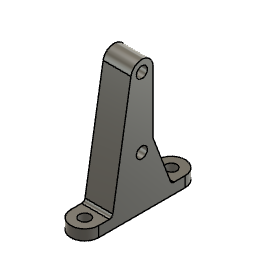
VL53L0X_Mount v9 (Autodesk Fusion 360 design; units mm, degrees)
Autodesk Fusion 360 part; units mm, degrees
sketch "Skizze1" plane through (0, 0, 0) normal (0, 1, 0) x (1, 0, 0)
  circle A0 centre (0.1472, 12.45) radius 1.6
  circle A1 centre (0.1472, -12.45) radius 1.6
  line L0 (0, 0) -> (50, 0) construction
  line L1 (4.1472, 12.45) -> (4.1472, -12.45)
  line L2 (-3.8528, 12.45) -> (-3.8528, -12.45)
  arc A2 (4.1472, 12.45) -> (-3.8528, 12.45) centre (0.1472, 12.45) ccw
  arc A3 (-3.8528, -12.45) -> (4.1472, -12.45) centre (0.1472, -12.45) ccw
  dimension "d1" = 24.9
  dimension "d2" = 3.2
  dimension "d3" = 8
  constraint coincident L0.start origin
  constraint horizontal L0
  constraint symmetric A0 A1 L0
  constraint concentric A0 A2
  constraint concentric A1 A3
  constraint symmetric L0 A2 A3
  constraint tangent L1 A3
  constraint tangent L1 A2
  constraint tangent L2 A3
  constraint vertical L2
  measures "d1" distance of A0.centre A1.centre
  measures "d2" diameter of A0
  measures "d3" diameter of A2
extrude "Extrusion1" add sketch "Skizze1" along normal blind 3
sketch "Skizze2" plane through (4.1472, 0, 0) normal (1, 0, 0) x (0, 0, -1)
  line L0 (-12.45, 0) -> (12.45, 0)
  line L1 (12.45, 0) -> (12.45, 3)
  line L2 (12.45, 3) -> (-12.45, 3)
  line L3 (-12.45, 3) -> (-12.45, 0)
  arc A0 (3.2, 35) -> (-3.1577, 35.5188) centre (0, 35) ccw
  line L4 (0, 0) -> (0, 43) construction
  circle A1 centre (0, 35) radius 1.6
  circle A2 centre (0, 15) radius 1.6
  line L5 (0, 25) -> (20, 25) construction
  line L6 (8.5, 3) -> (3.2, 17)
  line L7 (3.2, 17) -> (3.2, 35)
  line L8 (-3.1577, 35.5188) -> (-8.5, 3)
  dimension "d7" = 25
  dimension "d8" = 3.2
  dimension "d9" = 20
  dimension "d10" = 3.2
  dimension "d17" = 8.5
  dimension "d18" = 14
  dimension "d19" = 8.5
  constraint coincident L4.start origin
  constraint perpendicular L0 L4
  constraint coincident A0.centre L4
  constraint concentric A0 A1
  constraint coincident L4 A2.centre
  constraint coincident L4 L5.start
  constraint perpendicular L4 L5
  constraint symmetric A1 A2 L5
  constraint coincident L2 L6.start
  constraint tangent A0 L7
  constraint coincident L2 L8.end
  constraint tangent A0 L8
  constraint vertical L7
  measures "d7" distance of L4.start L5
  measures "d8" diameter of A1
  measures "d9" distance of A0.centre A2.centre
  measures "d10" radius of A0
  measures "d17" horizontal distance of L4.start L6.start
  measures "d18" vertical distance of L6.start L6.end
  measures "d19" horizontal distance of L4.start L8.end
extrude "Extrusion2" add sketch "Skizze2" against normal blind 8 contours L2 A0 L6 L7 L8
fillet "Abrundung3" radius 1 3 edges at (0.1472, 17, -3.2) (0.1472, 3, -8.5) (0.1472, 3, 8.5)
